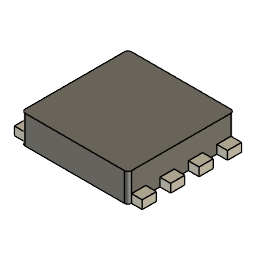
SKY13317-373LF (Autodesk Fusion 360 design; units mm, degrees)
Autodesk Fusion 360 part; units mm, degrees
sketch "草图1" plane through (0, 0, 0) normal (0, 0, 1) x (1, 0, 0)
  line L0 (-0.9, 0.7) -> (-0.6, 0.7)
  arc A0 (-0.55, 0.65) -> (-0.6, 0.7) centre (-0.6, 0.65) ccw
  line L1 (-0.55, 0.65) -> (-0.55, 0.55)
  arc A1 (-0.6, 0.5) -> (-0.55, 0.55) centre (-0.6, 0.55) ccw
  line L2 (-0.6, 0.5) -> (-0.9, 0.5)
  line L3 (-0.9, 0.5) -> (-0.9, 0.7)
  line L4 (0, 2.2) -> (0, -1) construction
  line L5 (-2.7, 0) -> (2.5608, 0) construction
  line L6 (-1.4896, 0.4) -> (-0.5, 0.4) construction
  line L7 (-0.9, 0.1) -> (-0.6, 0.1)
  line L8 (-0.9, 0.3) -> (-0.9, 0.1)
  line L9 (-0.6, 0.3) -> (-0.9, 0.3)
  line L10 (-0.55, 0.15) -> (-0.55, 0.25)
  arc A2 (-0.6, 0.1) -> (-0.55, 0.15) centre (-0.6, 0.15) ccw
  arc A3 (-0.55, 0.25) -> (-0.6, 0.3) centre (-0.6, 0.25) ccw
  arc A4 (-0.6, -0.7) -> (-0.55, -0.65) centre (-0.6, -0.65) ccw
  line L11 (-0.6, -0.3) -> (-0.9, -0.3)
  line L12 (-0.9, -0.7) -> (-0.6, -0.7)
  line L13 (-0.55, -0.65) -> (-0.55, -0.55)
  line L14 (-0.9, -0.3) -> (-0.9, -0.1)
  arc A5 (-0.55, -0.55) -> (-0.6, -0.5) centre (-0.6, -0.55) ccw
  line L15 (-0.6, -0.5) -> (-0.9, -0.5)
  line L16 (-0.55, -0.15) -> (-0.55, -0.25)
  arc A6 (-0.55, -0.15) -> (-0.6, -0.1) centre (-0.6, -0.15) ccw
  arc A7 (-0.6, -0.3) -> (-0.55, -0.25) centre (-0.6, -0.25) ccw
  line L17 (-0.9, -0.1) -> (-0.6, -0.1)
  line L18 (-0.9, -0.5) -> (-0.9, -0.7)
  arc A8 (0.6, -0.5) -> (0.55, -0.55) centre (0.6, -0.55) ccw
  line L19 (0.55, -0.65) -> (0.55, -0.55)
  arc A9 (0.6, -0.1) -> (0.55, -0.15) centre (0.6, -0.15) ccw
  line L20 (0.9, -0.5) -> (0.9, -0.7)
  line L21 (0.6, -0.5) -> (0.9, -0.5)
  arc A10 (0.55, -0.65) -> (0.6, -0.7) centre (0.6, -0.65) ccw
  line L22 (0.9, -0.7) -> (0.6, -0.7)
  line L23 (0.6, -0.3) -> (0.9, -0.3)
  line L24 (0.9, -0.3) -> (0.9, -0.1)
  line L25 (0.9, -0.1) -> (0.6, -0.1)
  line L26 (0.55, -0.15) -> (0.55, -0.25)
  arc A11 (0.55, -0.25) -> (0.6, -0.3) centre (0.6, -0.25) ccw
  line L27 (0.6, 0.3) -> (0.9, 0.3)
  line L28 (0.9, 0.1) -> (0.6, 0.1)
  line L29 (0.9, 0.3) -> (0.9, 0.1)
  arc A12 (0.55, 0.15) -> (0.6, 0.1) centre (0.6, 0.15) ccw
  arc A13 (0.6, 0.3) -> (0.55, 0.25) centre (0.6, 0.25) ccw
  line L30 (0.55, 0.15) -> (0.55, 0.25)
  arc A14 (0.6, 0.7) -> (0.55, 0.65) centre (0.6, 0.65) ccw
  line L31 (0.6, 0.5) -> (0.9, 0.5)
  line L32 (0.9, 0.7) -> (0.6, 0.7)
  arc A15 (0.55, 0.55) -> (0.6, 0.5) centre (0.6, 0.55) ccw
  line L33 (0.9, 0.5) -> (0.9, 0.7)
  line L34 (0.55, 0.65) -> (0.55, 0.55)
  line L35 (-0.2, 0.6) -> (-0.35, 0.45)
  line L36 (-0.35, 0.45) -> (-0.35, -0.5522)
  arc A16 (-0.35, -0.5522) -> (-0.3146, -0.6) centre (-0.3, -0.5522) ccw
  line L37 (-0.3146, -0.6) -> (-0.1, -0.6)
  line L38 (-0.1, -0.6) -> (-0.1, -0.65)
  line L39 (-0.1, -0.65) -> (0.1, -0.65)
  line L40 (0.1, -0.65) -> (0.1, -0.6)
  line L41 (0.1, -0.6) -> (0.3, -0.6)
  arc A17 (0.3, -0.6) -> (0.35, -0.55) centre (0.3, -0.55) ccw
  line L42 (0.35, -0.55) -> (0.35, 0.5543)
  arc A18 (0.35, 0.5543) -> (0.3202, 0.6) centre (0.3, 0.5543) ccw
  line L43 (0.3202, 0.6) -> (0.1, 0.6)
  line L44 (0.1, 0.6) -> (0.1, 0.65)
  line L45 (0.1, 0.65) -> (-0.1, 0.65)
  line L46 (-0.1, 0.65) -> (-0.1, 0.6)
  line L47 (-0.1, 0.6) -> (-0.2, 0.6)
  line L48 (-0.7, 0.75) -> (0.7, 0.75)
  arc A19 (0.75, 0.7) -> (0.7, 0.75) centre (0.7, 0.7) ccw
  line L49 (0.75, 0.7) -> (0.75, -0.7)
  arc A20 (0.7, -0.75) -> (0.75, -0.7) centre (0.7, -0.7) ccw
  line L50 (0.7, -0.75) -> (-0.7, -0.75)
  arc A21 (-0.75, -0.7) -> (-0.7, -0.75) centre (-0.7, -0.7) ccw
  line L51 (-0.75, -0.7) -> (-0.75, 0.7)
  arc A22 (-0.7, 0.75) -> (-0.75, 0.7) centre (-0.7, 0.7) ccw
  dimension "d1" = 0.2
  dimension "d2" = 0.35
  dimension "d3" = 0.05
  dimension "d4" = 0.55
  dimension "d5" = 0.5
  dimension "d6" = 0.4
  dimension "d7" = 0.05
  dimension "d8" = 0.2
  dimension "d9" = 0.2
  dimension "d10" = 0.7
  dimension "d11" = 0.05
  dimension "d12" = 0.05
  dimension "d14" = 0.15
  dimension "d15" = 0.15
  dimension "d16" = 1.2
  dimension "d17" = 0.05
  dimension "d18" = 1.5
  dimension "d19" = 1.5
  constraint horizontal L0
  constraint tangent L0 A0
  constraint perpendicular L0 L1
  constraint tangent L1 A1
  constraint tangent A1 L2
  constraint tangent A0 L1
  constraint equal A0 A1
  constraint perpendicular L2 L3
  constraint parallel L0 L2
  constraint vertical L4
  constraint horizontal L5
  constraint parallel L5 L6
  constraint symmetric L0.start L6 L7.start
  constraint symmetric L0.end L6 L7.end
  constraint symmetric A0.start L6 L10.start
  constraint symmetric A0 L6 A2
  constraint symmetric L1.end L6 L10.end
  constraint symmetric A1.start L6 L9.start
  constraint symmetric A1 L6 A3
  constraint symmetric L2.end L6 L8.start
  constraint symmetric L0.start L5 L12.start
  constraint symmetric L0.end L5 A4.start
  constraint symmetric A0.start L5 A4.end
  constraint symmetric A0 L5 A4
  constraint symmetric L1.end L5 L13.end
  constraint symmetric A1.start L5 A5.end
  constraint symmetric A1 L5 A5
  constraint symmetric L2.end L5 L15.end
  constraint symmetric L5 L9.start L11.start
  constraint symmetric L5 L7.end A6.end
  constraint symmetric L5 L8.start L11.end
  constraint symmetric L5 L7.start L14.end
  constraint symmetric L5 L10.start L16.start
  constraint symmetric L5 L10.end L16.end
  constraint symmetric L5 A2 A6
  constraint symmetric L5 A3 A7
  constraint symmetric L0.start L4 L32.start
  constraint symmetric L0.end L4 A14.start
  constraint symmetric A0.start L4 A14.end
  constraint symmetric A0 L4 A14
  constraint symmetric L1.end L4 A15.start
  constraint symmetric A1.start L4 L31.start
  constraint symmetric A1 L4 A15
  constraint symmetric L2.end L4 L31.end
  constraint symmetric L4 L9.start L27.start
  constraint symmetric L4 L7.end L28.end
  constraint symmetric L4 L8.start L27.end
  constraint symmetric L4 L7.start L28.start
  constraint symmetric L4 L10.start A12.start
  constraint symmetric L4 L10.end A13.end
  constraint symmetric L4 A2 A12
  constraint symmetric L4 A3 A13
  constraint symmetric L4 L16.start A9.end
  constraint symmetric L4 L16.end L26.end
  constraint symmetric L4 L12.start L20.end
  constraint symmetric L4 A4.start A10.end
  constraint symmetric L4 L11.end L23.end
  constraint symmetric L4 A4.end L19.start
  constraint symmetric L4 L13.end A8.end
  constraint symmetric L4 L15.end L20.start
  constraint symmetric L4 L14.end L24.end
  constraint symmetric L4 A6.end A9.start
  constraint symmetric L4 L11.start L23.start
  constraint symmetric L4 A5.end A8.start
  constraint symmetric L4 A4 A10
  constraint symmetric L4 A5 A8
  constraint symmetric L4 A6 A9
  constraint symmetric L4 A7 A11
  constraint perpendicular L2 L36
  constraint tangent L36 A16
  constraint perpendicular L36 L37
  constraint perpendicular L4 L39
  constraint perpendicular L4 L41
  constraint tangent L41 A17
  constraint tangent A17 L42
  constraint perpendicular L41 L42
  constraint tangent L42 A18
  constraint perpendicular L42 L43
  constraint perpendicular L43 L44
  constraint perpendicular L4 L45
  constraint perpendicular L43 L46
  constraint perpendicular L46 L47
  constraint equal A17 A18
  constraint equal A16 A17
  constraint parallel L4 L38
  constraint parallel L4 L40
  constraint symmetric L4 L38 L40
  constraint collinear L37 L41
  constraint collinear L43 L47
  constraint horizontal L48
  constraint tangent L48 A19
  constraint perpendicular L48 L49
  constraint tangent L49 A20
  constraint tangent L50 A21
  constraint tangent L51 A22
  constraint tangent L48 A22
  constraint tangent A19 L49
  constraint tangent A20 L50
  constraint tangent A21 L51
  constraint parallel L49 L51
  constraint parallel L48 L50
  constraint equal A19 A20
  constraint equal A20 A21
  constraint equal A21 A22
  constraint symmetric L4 L49 L51
  constraint symmetric L5 L48 L50
  measures "d1" distance of L0.start L2.end
  measures "d2" distance of L1 L3
  measures "d3" radius of A0
  measures "d4" distance of L1 L4
  measures "d5" distance of L2.end L5
  measures "d6" distance of L5 L6
  measures "d7" radius of A16
  measures "d8" distance of L38.end L39.end
  measures "d9" distance of L44.end L45.end
  measures "d10" distance of L36 L42
  measures "d11" distance of L43 L45
  measures "d12" distance of L39 L41
  measures "d14" horizontal distance of L35.start L35.end
  measures "d15" vertical distance of L35.start L35.end
  measures "d16" distance of L41 L43
  measures "d17" radius of A19
  measures "d18" distance of L48 L50
  measures "d19" distance of L49 L51
extrude "拉伸1" add sketch "草图1" along normal blind 0.4 contours L0 A0 L1 A1 L2 L7 L9 L10 A2 A3 A4 L11 L12 L13 A5 L15 L16 A6 A7 L17 A8 L19 A9 L21 A10 L22 L23 L25 L26 A11 L27 L28 A12 A13 L30 A14 L31 L32 A15 L34 L48 A19 L49 A20 L50 A21 L51 A22 | L0 A0 L1 A1 L2 L51 | L7 L9 L10 A2 A3 L51 | A14 L31 L32 A15 L34 L49 | L11 L16 A6 A7 L17 L51 | L27 L28 A12 A13 L30 L49 | A4 L12 L13 A5 L15 L51 | A9 L23 L25 L26 A11 L49 | A8 L19 L21 A10 L22 L49 | L35 L36 A16 L37 L38 L39 L40 L41 A17 L42 A18 L43 L44 L45 L46 L47 makes body 1
extrude "拉伸2" cut sketch "草图1" along normal blind 0.12 contours L0 L2 L3 L51 | L0 A0 L1 A1 L2 L51 | L7 L8 L9 L51 | L7 L9 L10 A2 A3 L51 | A14 L31 L32 A15 L34 L49 | L31 L32 L33 L49 | L11 L14 L17 L51 | L11 L16 A6 A7 L17 L51 | L27 L28 A12 A13 L30 L49 | L27 L28 L29 L49 | L12 L15 L18 L51 | A4 L12 L13 A5 L15 L51 | A9 L23 L25 L26 A11 L49 | L23 L24 L25 L49 | A8 L19 L21 A10 L22 L49 | L20 L21 L22 L49 | L35 L36 A16 L37 L38 L39 L40 L41 A17 L42 A18 L43 L44 L45 L46 L47 bodies 1
extrude "拉伸3" add sketch "草图1" along normal blind 0.12 separate body contours L0 L2 L3 L51 | L0 A0 L1 A1 L2 L51 | L7 L8 L9 L51 | L7 L9 L10 A2 A3 L51 | A14 L31 L32 A15 L34 L49 | L31 L32 L33 L49 | L11 L14 L17 L51 | L11 L16 A6 A7 L17 L51 | L27 L28 A12 A13 L30 L49 | L27 L28 L29 L49 | L12 L15 L18 L51 | A4 L12 L13 A5 L15 L51 | A9 L23 L25 L26 A11 L49 | L23 L24 L25 L49 | A8 L19 L21 A10 L22 L49 | L20 L21 L22 L49 | L35 L36 A16 L37 L38 L39 L40 L41 A17 L42 A18 L43 L44 L45 L46 L47 makes body 2 at (0.8, 0.1667, 0) makes body 3 at (-0.7, -0.2333, 0) makes body 4 at (-0.7, -0.6333, 0) makes body 5 at (0.8, 0.5667, 0) makes body 6 at (0.7, -0.1667, 0) makes body 7 at (-0.8, 0.2333, 0) makes body 8 at (-0.05, 0.15, 0) makes body 9 at (-0.8, 0.6333, 0) makes body 10 at (0.8, -0.6333, 0)
sketch "草图2" plane through (0, -0.7, 0) normal (0, -1, 0) x (1, 0, 0)
  line L0 (-0.9, 0) -> (-0.6, 0)
  line L1 (-0.6, 0) -> (-0.6, 0.12)
  line L2 (-0.6, 0.12) -> (-0.9, 0.12)
  line L3 (-0.9, 0.12) -> (-0.9, 0)
